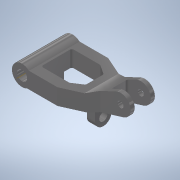
# Autodesk Inventor part: wheel_holder
Saved by Autodesk Inventor 2020 (Build 240168000, 168)
## iProperties
Created: 2015-12-05
Part Number: wheel_holder
Material: Acero inoxidable, austenítico
Document SubType Name: Modeling
Designer: MIGUEL ANGEL
Density: 8 g/cm^3
Appearance: Semipulido
Author: MIGUEL ANGEL
Autodesk Inventor part; units mm, degrees
sketch "Boceto1" plane through (0, 0, 0) normal (0, 1, 0) x (-1, 0, 0)
  circle A0 centre (0, 0) radius 10
  line L0 (-4.9878, -8.6673) -> (-54.9878, -8.6673)
  line L1 (-6.7993, 7.3327) -> (-53.4848, 7.3327)
  line L2 (-54.9878, -8.6673) -> (-87.1955, 1.2044)
  arc A1 (-81.3346, 20.3264) -> (-87.1955, 1.2044) centre (-84.2651, 10.7654) ccw
  line L3 (-81.3346, 20.3264) -> (-53.4848, 7.3327)
  dimension "d0" = 20
  dimension "d1" = 16
  dimension "d2" = 10
  dimension "d3" = 50
  dimension "d25" = 154.988
  constraints: 8 end point, 4 point on circle, 2 centre point, 2 horizontal, 1 coincident, 1 tangent
  measures "d0" diameter of A0
  measures "d1" distance between parallel lines of L1 L0
  measures "d2" radius of A1
  measures "d3" distance of L0.start L0.end
  measures "d25" angle of L3 L1
extrude "Extrusión1" add sketch "Boceto1" along normal blind 50
sketch "Boceto2" plane through (54.9878, 0, -8.6673) normal (0, 0, -1) x (-1, 0, 0)
  line L0 (-39.2772, 0) -> (-39.2772, 50) projected
  line L1 (-32.2077, 50) -> (0, 50) projected
  line L2 (-32.2077, 0) -> (0, 0) projected
  line L3 (0, 0) -> (50, 0) projected
  line L4 (0, 50) -> (50, 50) projected
  line L5 (92.4078, 25) -> (-89.4019, 25)
  line L6 (-39.2772, 17) -> (-18.1038, 17)
  line L7 (-16.1038, 19) -> (-16.1038, 25)
  line L8 (-39.2772, 13) -> (-9.2772, 13)
  line L9 (-9.2772, 13) -> (20, 0)
  line L10 (48.1885, 0) -> (1.503, 0) projected
  line L11 (8.207, 25) -> (8.207, 17.2439)
  line L12 (9.1152, 15.5682) -> (17.5023, 10.1036)
  line L13 (18.5941, 9.7793) -> (44, 9.7793)
  line L14 (46, 11.7793) -> (46, 25)
  line L15 (50, 0) -> (20, 0)
  line L16 (64.9878, 0) -> (48.1885, 0) projected
  line L17 (50, 50) -> (50, 0) projected
  arc A0 (-18.1038, 17) -> (-16.1038, 19) centre (-18.1038, 19) ccw
  arc A1 (8.207, 17.2439) -> (9.1152, 15.5682) centre (10.207, 17.2439) ccw
  arc A2 (17.5023, 10.1036) -> (18.5941, 9.7793) centre (18.5941, 11.7793) ccw
  arc A3 (44, 9.7793) -> (46, 11.7793) centre (44, 11.7793) ccw
  line L18 (20, 0) -> (-39.2772, 0)
  line L19 (-26.3468, 0) -> (-39.2772, 0) projected
  line L20 (-39.2772, 17) -> (-39.2772, 25)
  line L21 (0, 50) -> (50, 50)
  line L22 (-39.2772, 33) -> (-18.1038, 33)
  line L23 (-16.1038, 31) -> (-16.1038, 25)
  line L24 (-39.2772, 37) -> (-9.2772, 37)
  line L25 (-9.2772, 37) -> (20, 50)
  line L26 (48.1885, 50) -> (1.503, 50)
  line L27 (8.207, 25) -> (8.207, 32.7561)
  line L28 (9.1152, 34.4318) -> (17.5023, 39.8964)
  line L29 (18.5941, 40.2207) -> (44, 40.2207)
  line L30 (46, 38.2207) -> (46, 25)
  line L31 (50, 0) -> (50, 50)
  arc A4 (-16.1038, 31) -> (-18.1038, 33) centre (-18.1038, 31) ccw
  arc A5 (9.1152, 34.4318) -> (8.207, 32.7561) centre (10.207, 32.7561) ccw
  arc A6 (18.5941, 40.2207) -> (17.5023, 39.8964) centre (18.5941, 38.2207) ccw
  arc A7 (46, 38.2207) -> (44, 40.2207) centre (44, 38.2207) ccw
  line L32 (20, 50) -> (-39.2772, 50)
  line L33 (-39.2772, 50) -> (-39.2772, 37)
  line L34 (-39.2772, 33) -> (-39.2772, 17)
  line L35 (-39.2772, 13) -> (-39.2772, 0)
  point P0 (54.9878, 0)
  point P1 (1.503, 25)
  point P2 (18, 9.7793)
  point P3 (46, 9.7793)
  dimension "d6" = 12
  dimension "d7" = 4
  dimension "d8" = 30
  dimension "d9" = 30
  dimension "d10" = 28
  dimension "d11" = 4
  dimension "d12" = 2
  constraints: 54 end point, 22 symmetric about line, 16 point on circle, 11 point on line, 8 centre point, 8 tangent, 4 perpendicular, 3 collinear, 3 equal radius, 2 horizontal, 2 midpoint, 1 horizontal alignment, 1 vertical, 1 vertical alignment, 4 other
  measures "d6" distance of L20.end L8.start
  measures "d7" distance between parallel lines of L6 L8
  measures "d8" distance of L3.end L9.end
  measures "d9" distance of L8.start L8.end
  measures "d10" distance of point (18, 9.779) point (46, 9.779)
  measures "d11" distance between parallel lines of L17 L14
  measures "d12" radius of A0
extrude "Extrusión2" cut sketch "Boceto2" against normal through all contours L0 L8 L9 L3 L2 L18 | L0 L5 L7 A0 L6 | L0 L22 A4 L23 L5 | L0 L32 L1 L4 L25 L24 | L27 A5 L28 A6 L29 A7 L30 L5 | L5 L14 A3 L13 A2 L12 A1 L11
sketch "Boceto3" plane through (0, 50, 0) normal (0, 1, 0) x (1, 0, 0)
  circle A0 centre (0, 0) radius 5
  arc A1 (81.3346, -20.3264) -> (87.1955, -1.2044) centre (84.2651, -10.7654) ccw projected
  circle A2 centre (84.2651, -10.7654) radius 3
  dimension "d15" = 10
  dimension "d16" = 6
  constraints: 2 centre point, 2 coincident
  measures "d15" diameter of A0
  measures "d16" diameter of A2
extrude "Extrusión3" cut sketch "Boceto3" against normal through all
sketch "Boceto4" plane through (4.9878, 0, -8.6673) normal (0, 0, -1) x (-1, 0, 0)
  line L0 (-50, 8.8806) -> (-50, 41.1194) projected
  line L1 (-41.793, 17.2439) -> (-50, 17.2439)
  line L2 (-50, 17.2439) -> (-50, 33.3843)
  line L3 (-50, 33.3843) -> (-41.793, 33.3843)
  line L4 (-41.793, 33.3843) -> (-41.793, 17.2439)
  point P0 (4.9878, 0)
  constraints: 8 end point, 2 parallel, 1 horizontal, 1 perpendicular, 1 point on line
extrude "Extrusión4" add sketch "Boceto4" along normal blind 20
sketch "Boceto5" plane through (54.9878, 17.2439, -8.6673) normal (1, 0, 0) x (0, 0, -1)
  line L0 (20, 16.1404) -> (20, 0) projected
  line L1 (0, 16.1404) -> (20, 16.1404) projected
  line L2 (0, 0) -> (20, 0) projected
  circle A0 centre (11.9298, 8.0702) radius 8.0702
  line L3 (11.9298, 16.1404) -> (20, 16.1404)
  line L4 (20, 16.1404) -> (20, 8.0702)
  line L5 (20, 8.0702) -> (20, 0)
  line L6 (20, 0) -> (11.9298, 0)
  circle A1 centre (11.9298, 8.0702) radius 4
  point P0 (-8.6673, -17.2439)
  dimension "d21" = 8
  constraints: 8 end point, 5 tangent, 3 point on circle, 2 centre point, 2 collinear, 2 point on line, 1 coincident, 1 midpoint
  measures "d21" diameter of A1
extrude "Extrusión5" cut sketch "Boceto5" against normal up to next contours L0 A0 L1 | L0 L2 A0 | A1
ref_plane "Plano de trabajo1" through (54.9878, 17.2439, -20.5971) normal (1, 0, 0) x (0, 0, -1)
ref_plane "Plano de trabajo3" through (27.4939, 50, 0) normal (1, 0, 0) x (0, -1, 0)
ref_plane "Plano de trabajo2" through (0, 50, 0) normal (1, 0, 0) x (0, -1, 0)
mirror "Simetría1" about plane through (27.4939, 50, 0) normal (1, 0, 0) of "Extrusión5", "Extrusión4"
ref_plane "Plano de trabajo6" through (46.7808, 33.3843, -20.5971) normal (-1, 0, 0) x (0, 0, 1)
